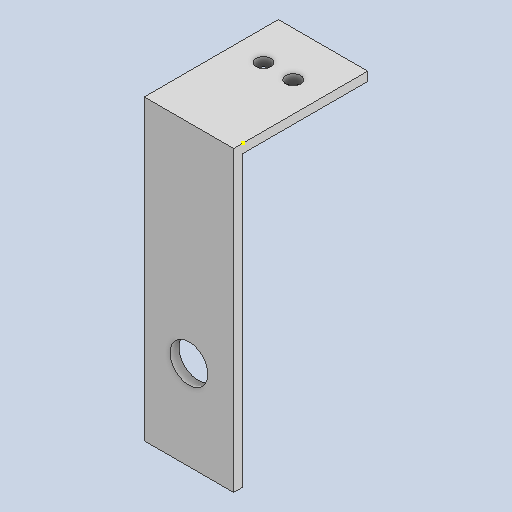
# Autodesk Inventor part: Angle
Saved by Autodesk Inventor 2024 (Build 280153000, 153)
## iProperties
Created: 2024-02-05
Part Number: Angle
Material: Generic
Document SubType Name: Modeling
Designer: Ramji Yadav
Density: 1 g/cm^3
Appearance: Default
Author: Ramji Yadav
Autodesk Inventor part; units mm, degrees
ref_plane "YZ Plane" through (0, 0, 0) normal (1, 0, 0) x (0, 1, 0)
ref_plane "XZ Plane" through (0, 0, 0) normal (0, 1, 0) x (-1, 0, 0)
ref_plane "XY Plane" through (0, 0, 0) normal (0, 0, 1) x (1, 0, 0)
sketch "Sketch1" plane through (0, 0, 0) normal (0, 0, 1) x (1, 0, 0)
  line L0 (0, 0) -> (-30, 0)
  line L1 (-30, 0) -> (-30, 8)
  line L2 (-30, 8) -> (0, 8)
  line L3 (0, 8) -> (0, 0)
  line L4 (0, 8) -> (-30, 8)
  line L5 (-30, 8) -> (-30, -92)
  line L6 (-30, -92) -> (0, -92)
  line L7 (0, -92) -> (0, 8)
  dimension "d0" = 30
  dimension "d1" = 8
  dimension "d2" = 100
  constraints: 16 end point, 4 parallel, 2 horizontal, 2 perpendicular
  measures "d0" distance of L1.end L2.end
  measures "d1" distance of L0.end L1.end
  measures "d2" distance of L5.end L4.end
extrude "Extrusion1" add sketch "Sketch1" along normal blind 3
sketch "Sketch2" plane through (0, 0, 0) normal (0, 0, -1) x (-1, 0, 0)
  line L0 (30, 8) -> (30, -92) projected
  line L1 (0, -92) -> (0, 8) projected
  line L2 (30, 8) -> (0, 8)
  line L3 (0, 8) -> (0, 5)
  line L4 (0, 5) -> (30, 5)
  line L5 (30, 5) -> (30, 8)
  point P0 (0, 0)
  point P1 (0, 8)
  dimension "d5" = 3
  constraints: 8 end point, 2 parallel, 1 horizontal, 1 perpendicular, 1 point on line
  measures "d5" distance of L3.end L2.end
extrude "Extrusion2" add sketch "Sketch2" along normal blind 42
sketch "Sketch3" plane through (-30, 8, 3) normal (0, 1, 0) x (1, 0, 0)
  line L0 (0, 45) -> (0, 0) projected
  line L1 (0, 45) -> (0, 30)
  line L2 (0, 30) -> (10, 30)
  circle A0 centre (10, 30) radius 2.5
  line L3 (30, 0) -> (30, 45) projected
  line L4 (30, 45) -> (30, 30)
  circle A1 centre (20, 30) radius 2.5
  point P0 (30, 3)
  dimension "d8" = 15
  dimension "d9" = 10
  dimension "d10" = 5
  dimension "d11" = 15
  dimension "d12" = 5
  dimension "d13" = 10
  constraints: 6 end point, 3 point on line, 2 centre point, 1 coincident, 1 horizontal
  measures "d8" distance of L0.start L1.end
  measures "d9" distance of L1.end L2.end
  measures "d10" diameter of A0
  measures "d11" distance of L3.end L4.end
  measures "d12" diameter of A1
  measures "d13" distance of A1.centre L2.end
extrude "Extrusion3" cut sketch "Sketch3" against normal blind 42
sketch "Sketch4" plane through (0, 0, 0) normal (0, 0, -1) x (-1, 0, 0)
  circle A0 centre (15, -62) radius 6.35
  line L0 (30, -92) -> (0, -92) projected
  line L1 (0, -92) -> (0, 5) projected
  point P0 (0, 0)
  dimension "d16" = 12.7
  dimension "d17" = 30
  dimension "d18" = 15
  constraints: 1 centre point
  measures "d16" diameter of A0
  measures "d17" distance from line of L0 A0.centre
  measures "d18" distance from line of L1 A0.centre
extrude "Extrusion4" cut sketch "Sketch4" against normal blind 42
sketch "Sketch5" plane through (-30, 8, 3) normal (0, 1, 0) x (1, 0, 0)
  point P0 (30, 3)
sketch "Sketch6" plane through (-30, 8, 3) normal (0, 1, 0) x (1, 0, 0)
  point P0 (30, 3)
body "Solid1"
